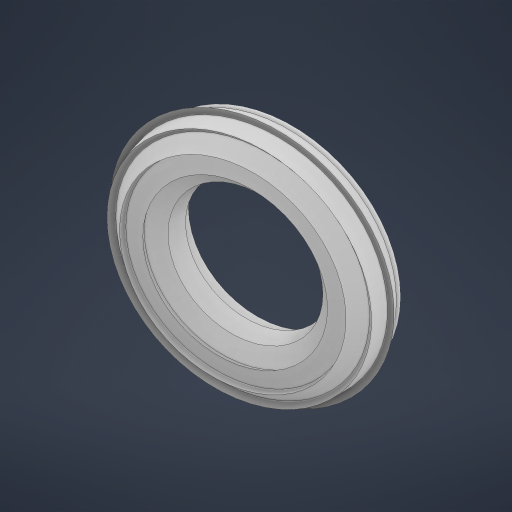
# Autodesk Inventor part: coba
Saved by Autodesk Inventor 2024.3 (Build 283343000, 343)
## iProperties
Created: 2025-06-21
Part Number: coba
Material: Generic
Document SubType Name: Modeling
Designer: Akbar Syihabuddin
Density: 1 g/cm^3
Appearance: Default
Author: Akbar Syihabuddin
Autodesk Inventor part; units mm, degrees
ref_plane "YZ Plane" through (0, 0, 0) normal (1, 0, 0) x (0, 1, 0)
ref_plane "XZ Plane" through (0, 0, 0) normal (0, 1, 0) x (-1, 0, 0)
ref_plane "XY Plane" through (0, 0, 0) normal (0, 0, 1) x (1, 0, 0)
sketch "Sketch1" plane through (0, 0, 0) normal (0, 1, 0) x (-1, 0, 0)
  line L0 (0, 1270.9169) -> (0, 1070.9169)
  line L1 (0, 1070.9169) -> (280.5773, 1070.9169)
  circle A0 centre (280.5773, 1070.9169) radius 150
  arc A1 (0, 862.6395) -> (280.5773, 1070.9169) centre (285.6481, 770.9597) ccw
  line L2 (0, 1671.4874) -> (1000, 1671.4874)
  line L3 (1000, 1671.4874) -> (1000, 2371.4874)
  line L4 (1000, 2371.4874) -> (0, 2371.4874)
  line L5 (0, 2371.4874) -> (0, 1671.4874)
  line L6 (663.7557, 3727.8622) -> (677.7261, 3727.8622) construction
  line L7 (677.7261, 3727.8622) -> (677.7261, 3724.6141) construction
  line L8 (677.7261, 3724.6141) -> (663.7557, 3724.6141) construction
  line L9 (663.7557, 3724.6141) -> (663.7557, 3727.8622) construction
  line L10 (500, 2021.4874) -> (1196.7714, 1270.9169)
  line L11 (1196.7714, 1270.9169) -> (1168.0077, -285.8687)
  line L12 (1168.0077, -285.8687) -> (464.4615, -168.1988)
  line L13 (464.4615, -168.1988) -> (320.7847, -408.7683)
  line L14 (1361.4266, 1423.77) -> (-428.0148, 1423.77)
  line L15 (-500, 1671.4874) -> (-500, 2371.4874)
  line L16 (-500, 2371.4874) -> (-1500, 2371.4874)
  line L17 (-1500, 2371.4874) -> (-1500, 1671.4874)
  line L18 (-1500, 1671.4874) -> (-500, 1671.4874)
  line L19 (2500, 1671.4874) -> (2500, 2371.4874)
  line L20 (2500, 2371.4874) -> (1500, 2371.4874)
  line L21 (1500, 2371.4874) -> (1500, 1671.4874)
  line L22 (1500, 1671.4874) -> (2500, 1671.4874)
  line L23 (1000, 1671.4874) -> (1000, 2371.4874)
  line L24 (1000, 2371.4874) -> (0, 2371.4874)
  line L25 (0, 2371.4874) -> (0, 1671.4874)
  line L26 (0, 1671.4874) -> (1000, 1671.4874)
  line L27 (500, 2021.4874) -> (500, -515.8022)
  line L28 (1000, 871.4874) -> (0, 871.4874)
  line L29 (1000, 871.4874) -> (0, 871.4874)
  line L30 (1000, 171.4874) -> (1000, 871.4874)
  line L31 (1000, 171.4874) -> (1000, 871.4874)
  line L32 (0, 871.4874) -> (0, 171.4874)
  line L33 (0, 871.4874) -> (0, 171.4874)
  line L34 (0, 171.4874) -> (1000, 171.4874)
  line L35 (0, 171.4874) -> (1000, 171.4874)
  line L36 (1000, -628.5126) -> (0, -628.5126)
  line L37 (1000, -628.5126) -> (0, -628.5126)
  line L38 (1000, -1328.5126) -> (1000, -628.5126)
  line L39 (1000, -1328.5126) -> (1000, -628.5126)
  line L40 (0, -628.5126) -> (0, -1328.5126)
  line L41 (0, -628.5126) -> (0, -1328.5126)
  line L42 (0, -1328.5126) -> (1000, -1328.5126)
  line L43 (0, -1328.5126) -> (1000, -1328.5126)
  line L44 (1000, -2128.5126) -> (0, -2128.5126)
  line L45 (1000, -2128.5126) -> (0, -2128.5126)
  line L46 (1000, -2828.5126) -> (1000, -2128.5126)
  line L47 (1000, -2828.5126) -> (1000, -2128.5126)
  line L48 (0, -2128.5126) -> (0, -2828.5126)
  line L49 (0, -2128.5126) -> (0, -2828.5126)
  line L50 (0, -2828.5126) -> (1000, -2828.5126)
  line L51 (0, -2828.5126) -> (1000, -2828.5126)
  line L52 (1000, -3628.5126) -> (0, -3628.5126)
  line L53 (1000, -3628.5126) -> (0, -3628.5126)
  line L54 (1000, -4328.5126) -> (1000, -3628.5126)
  line L55 (1000, -4328.5126) -> (1000, -3628.5126)
  line L56 (0, -3628.5126) -> (0, -4328.5126)
  line L57 (0, -3628.5126) -> (0, -4328.5126)
  line L58 (0, -4328.5126) -> (1000, -4328.5126)
  line L59 (0, -4328.5126) -> (1000, -4328.5126)
  line L60 (1000, -5128.5126) -> (0, -5128.5126)
  line L61 (1000, -5128.5126) -> (0, -5128.5126)
  line L62 (1000, -5828.5126) -> (1000, -5128.5126)
  line L63 (1000, -5828.5126) -> (1000, -5128.5126)
  line L64 (0, -5128.5126) -> (0, -5828.5126)
  line L65 (0, -5128.5126) -> (0, -5828.5126)
  line L66 (0, -5828.5126) -> (1000, -5828.5126)
  line L67 (0, -5828.5126) -> (1000, -5828.5126)
  line L68 (1000, -6628.5126) -> (0, -6628.5126)
  line L69 (1000, -6628.5126) -> (0, -6628.5126)
  line L70 (1000, -7328.5126) -> (1000, -6628.5126)
  line L71 (1000, -7328.5126) -> (1000, -6628.5126)
  line L72 (0, -6628.5126) -> (0, -7328.5126)
  line L73 (0, -6628.5126) -> (0, -7328.5126)
  line L74 (0, -7328.5126) -> (1000, -7328.5126)
  line L75 (0, -7328.5126) -> (1000, -7328.5126)
  line L76 (1000, -8128.5126) -> (0, -8128.5126)
  line L77 (1000, -8128.5126) -> (0, -8128.5126)
  line L78 (1000, -8828.5126) -> (1000, -8128.5126)
  line L79 (1000, -8828.5126) -> (1000, -8128.5126)
  line L80 (0, -8128.5126) -> (0, -8828.5126)
  line L81 (0, -8128.5126) -> (0, -8828.5126)
  line L82 (0, -8828.5126) -> (1000, -8828.5126)
  line L83 (0, -8828.5126) -> (1000, -8828.5126)
  line L84 (1000, -9628.5126) -> (0, -9628.5126)
  line L85 (1000, -9628.5126) -> (0, -9628.5126)
  line L86 (1000, -10328.5126) -> (1000, -9628.5126)
  line L87 (1000, -10328.5126) -> (1000, -9628.5126)
  line L88 (0, -9628.5126) -> (0, -10328.5126)
  line L89 (0, -9628.5126) -> (0, -10328.5126)
  line L90 (0, -10328.5126) -> (1000, -10328.5126)
  line L91 (0, -10328.5126) -> (1000, -10328.5126)
  line L92 (1000, -11128.5126) -> (0, -11128.5126)
  line L93 (1000, -11128.5126) -> (0, -11128.5126)
  line L94 (1000, -11828.5126) -> (1000, -11128.5126)
  line L95 (1000, -11828.5126) -> (1000, -11128.5126)
  line L96 (0, -11128.5126) -> (0, -11828.5126)
  line L97 (0, -11128.5126) -> (0, -11828.5126)
  line L98 (0, -11828.5126) -> (1000, -11828.5126)
  line L99 (0, -11828.5126) -> (1000, -11828.5126)
  line L100 (1000, -12628.5126) -> (0, -12628.5126)
  line L101 (1000, -12628.5126) -> (0, -12628.5126)
  line L102 (1000, -13328.5126) -> (1000, -12628.5126)
  line L103 (1000, -13328.5126) -> (1000, -12628.5126)
  line L104 (0, -12628.5126) -> (0, -13328.5126)
  line L105 (0, -12628.5126) -> (0, -13328.5126)
  line L106 (0, -13328.5126) -> (1000, -13328.5126)
  line L107 (0, -13328.5126) -> (1000, -13328.5126)
  line L108 (1000, -14128.5126) -> (0, -14128.5126)
  line L109 (1000, -14128.5126) -> (0, -14128.5126)
  line L110 (1000, -14828.5126) -> (1000, -14128.5126)
  line L111 (1000, -14828.5126) -> (1000, -14128.5126)
  line L112 (0, -14128.5126) -> (0, -14828.5126)
  line L113 (0, -14128.5126) -> (0, -14828.5126)
  line L114 (0, -14828.5126) -> (1000, -14828.5126)
  line L115 (0, -14828.5126) -> (1000, -14828.5126)
  line L116 (1000, -15628.5126) -> (0, -15628.5126)
  line L117 (1000, -15628.5126) -> (0, -15628.5126)
  line L118 (1000, -16328.5126) -> (1000, -15628.5126)
  line L119 (1000, -16328.5126) -> (1000, -15628.5126)
  line L120 (0, -15628.5126) -> (0, -16328.5126)
  line L121 (0, -15628.5126) -> (0, -16328.5126)
  line L122 (0, -16328.5126) -> (1000, -16328.5126)
  line L123 (0, -16328.5126) -> (1000, -16328.5126)
  line L124 (1000, -17128.5126) -> (0, -17128.5126)
  line L125 (1000, -17128.5126) -> (0, -17128.5126)
  line L126 (1000, -17828.5126) -> (1000, -17128.5126)
  line L127 (1000, -17828.5126) -> (1000, -17128.5126)
  line L128 (0, -17128.5126) -> (0, -17828.5126)
  line L129 (0, -17128.5126) -> (0, -17828.5126)
  line L130 (0, -17828.5126) -> (1000, -17828.5126)
  line L131 (0, -17828.5126) -> (1000, -17828.5126)
  line L132 (1000, -18628.5126) -> (0, -18628.5126)
  line L133 (1000, -18628.5126) -> (0, -18628.5126)
  line L134 (1000, -19328.5126) -> (1000, -18628.5126)
  line L135 (1000, -19328.5126) -> (1000, -18628.5126)
  line L136 (0, -18628.5126) -> (0, -19328.5126)
  line L137 (0, -18628.5126) -> (0, -19328.5126)
  line L138 (0, -19328.5126) -> (1000, -19328.5126)
  line L139 (0, -19328.5126) -> (1000, -19328.5126)
  line L140 (1000, -20128.5126) -> (0, -20128.5126)
  line L141 (1000, -20128.5126) -> (0, -20128.5126)
  line L142 (1000, -20828.5126) -> (1000, -20128.5126)
  line L143 (1000, -20828.5126) -> (1000, -20128.5126)
  line L144 (0, -20128.5126) -> (0, -20828.5126)
  line L145 (0, -20128.5126) -> (0, -20828.5126)
  line L146 (0, -20828.5126) -> (1000, -20828.5126)
  line L147 (0, -20828.5126) -> (1000, -20828.5126)
  line L148 (1000, -21628.5126) -> (0, -21628.5126)
  line L149 (1000, -21628.5126) -> (0, -21628.5126)
  line L150 (1000, -22328.5126) -> (1000, -21628.5126)
  line L151 (1000, -22328.5126) -> (1000, -21628.5126)
  line L152 (0, -21628.5126) -> (0, -22328.5126)
  line L153 (0, -21628.5126) -> (0, -22328.5126)
  line L154 (0, -22328.5126) -> (1000, -22328.5126)
  line L155 (0, -22328.5126) -> (1000, -22328.5126)
  line L156 (1000, -23128.5126) -> (0, -23128.5126)
  line L157 (1000, -23128.5126) -> (0, -23128.5126)
  line L158 (1000, -23828.5126) -> (1000, -23128.5126)
  line L159 (1000, -23828.5126) -> (1000, -23128.5126)
  line L160 (0, -23128.5126) -> (0, -23828.5126)
  line L161 (0, -23128.5126) -> (0, -23828.5126)
  line L162 (0, -23828.5126) -> (1000, -23828.5126)
  line L163 (0, -23828.5126) -> (1000, -23828.5126)
  line L164 (1000, -24628.5126) -> (0, -24628.5126)
  line L165 (1000, -24628.5126) -> (0, -24628.5126)
  line L166 (1000, -25328.5126) -> (1000, -24628.5126)
  line L167 (1000, -25328.5126) -> (1000, -24628.5126)
  line L168 (0, -24628.5126) -> (0, -25328.5126)
  line L169 (0, -24628.5126) -> (0, -25328.5126)
  line L170 (0, -25328.5126) -> (1000, -25328.5126)
  line L171 (0, -25328.5126) -> (1000, -25328.5126)
  line L172 (1000, -26128.5126) -> (0, -26128.5126)
  line L173 (1000, -26128.5126) -> (0, -26128.5126)
  line L174 (1000, -26828.5126) -> (1000, -26128.5126)
  line L175 (1000, -26828.5126) -> (1000, -26128.5126)
  line L176 (0, -26128.5126) -> (0, -26828.5126)
  line L177 (0, -26128.5126) -> (0, -26828.5126)
  line L178 (0, -26828.5126) -> (1000, -26828.5126)
  line L179 (0, -26828.5126) -> (1000, -26828.5126)
  line L180 (1000, -27628.5126) -> (0, -27628.5126)
  line L181 (1000, -27628.5126) -> (0, -27628.5126)
  line L182 (1000, -28328.5126) -> (1000, -27628.5126)
  line L183 (1000, -28328.5126) -> (1000, -27628.5126)
  line L184 (0, -27628.5126) -> (0, -28328.5126)
  line L185 (0, -27628.5126) -> (0, -28328.5126)
  line L186 (0, -28328.5126) -> (1000, -28328.5126)
  line L187 (0, -28328.5126) -> (1000, -28328.5126)
  line L188 (1000, -29128.5126) -> (0, -29128.5126)
  line L189 (1000, -29128.5126) -> (0, -29128.5126)
  line L190 (1000, -29828.5126) -> (1000, -29128.5126)
  line L191 (1000, -29828.5126) -> (1000, -29128.5126)
  line L192 (0, -29128.5126) -> (0, -29828.5126)
  line L193 (0, -29128.5126) -> (0, -29828.5126)
  line L194 (0, -29828.5126) -> (1000, -29828.5126)
  line L195 (0, -29828.5126) -> (1000, -29828.5126)
  line L196 (1000, -30628.5126) -> (0, -30628.5126)
  line L197 (1000, -30628.5126) -> (0, -30628.5126)
  line L198 (1000, -31328.5126) -> (1000, -30628.5126)
  line L199 (1000, -31328.5126) -> (1000, -30628.5126)
  line L200 (0, -30628.5126) -> (0, -31328.5126)
  line L201 (0, -30628.5126) -> (0, -31328.5126)
  line L202 (0, -31328.5126) -> (1000, -31328.5126)
  line L203 (0, -31328.5126) -> (1000, -31328.5126)
  line L204 (1000, -32128.5126) -> (0, -32128.5126)
  line L205 (1000, -32128.5126) -> (0, -32128.5126)
  line L206 (1000, -32828.5126) -> (1000, -32128.5126)
  line L207 (1000, -32828.5126) -> (1000, -32128.5126)
  line L208 (0, -32128.5126) -> (0, -32828.5126)
  line L209 (0, -32128.5126) -> (0, -32828.5126)
  line L210 (0, -32828.5126) -> (1000, -32828.5126)
  line L211 (0, -32828.5126) -> (1000, -32828.5126)
  line L212 (1000, -33628.5126) -> (0, -33628.5126)
  line L213 (1000, -33628.5126) -> (0, -33628.5126)
  line L214 (1000, -34328.5126) -> (1000, -33628.5126)
  line L215 (1000, -34328.5126) -> (1000, -33628.5126)
  line L216 (0, -33628.5126) -> (0, -34328.5126)
  line L217 (0, -33628.5126) -> (0, -34328.5126)
  line L218 (0, -34328.5126) -> (1000, -34328.5126)
  line L219 (0, -34328.5126) -> (1000, -34328.5126)
  line L220 (1000, -35128.5126) -> (0, -35128.5126)
  line L221 (1000, -35128.5126) -> (0, -35128.5126)
  line L222 (1000, -35828.5126) -> (1000, -35128.5126)
  line L223 (1000, -35828.5126) -> (1000, -35128.5126)
  line L224 (0, -35128.5126) -> (0, -35828.5126)
  line L225 (0, -35128.5126) -> (0, -35828.5126)
  line L226 (0, -35828.5126) -> (1000, -35828.5126)
  line L227 (0, -35828.5126) -> (1000, -35828.5126)
  line L228 (1000, -36628.5126) -> (0, -36628.5126)
  line L229 (1000, -36628.5126) -> (0, -36628.5126)
  line L230 (1000, -37328.5126) -> (1000, -36628.5126)
  line L231 (1000, -37328.5126) -> (1000, -36628.5126)
  line L232 (0, -36628.5126) -> (0, -37328.5126)
  line L233 (0, -36628.5126) -> (0, -37328.5126)
  line L234 (0, -37328.5126) -> (1000, -37328.5126)
  line L235 (0, -37328.5126) -> (1000, -37328.5126)
  line L236 (1000, -38128.5126) -> (0, -38128.5126)
  line L237 (1000, -38128.5126) -> (0, -38128.5126)
  line L238 (1000, -38828.5126) -> (1000, -38128.5126)
  line L239 (1000, -38828.5126) -> (1000, -38128.5126)
  line L240 (0, -38128.5126) -> (0, -38828.5126)
  line L241 (0, -38128.5126) -> (0, -38828.5126)
  line L242 (0, -38828.5126) -> (1000, -38828.5126)
  line L243 (0, -38828.5126) -> (1000, -38828.5126)
  line L244 (1000, -39628.5126) -> (0, -39628.5126)
  line L245 (1000, -39628.5126) -> (0, -39628.5126)
  line L246 (1000, -40328.5126) -> (1000, -39628.5126)
  line L247 (1000, -40328.5126) -> (1000, -39628.5126)
  line L248 (0, -39628.5126) -> (0, -40328.5126)
  line L249 (0, -39628.5126) -> (0, -40328.5126)
  line L250 (0, -40328.5126) -> (1000, -40328.5126)
  line L251 (0, -40328.5126) -> (1000, -40328.5126)
  line L252 (1000, -41128.5126) -> (0, -41128.5126)
  line L253 (1000, -41128.5126) -> (0, -41128.5126)
  line L254 (1000, -41828.5126) -> (1000, -41128.5126)
  line L255 (1000, -41828.5126) -> (1000, -41128.5126)
  line L256 (0, -41128.5126) -> (0, -41828.5126)
  line L257 (0, -41128.5126) -> (0, -41828.5126)
  line L258 (0, -41828.5126) -> (1000, -41828.5126)
  line L259 (0, -41828.5126) -> (1000, -41828.5126)
  circle A2 centre (1648.4251, 5737.6204) radius 272.6746
  line L260 (1594.4602, 7563.1402) -> (599.9131, 7563.1402)
  line L261 (599.9131, 7563.1402) -> (599.9131, 6816.0626)
  line L262 (599.9131, 6816.0626) -> (1594.4602, 6816.0626)
  line L263 (1594.4602, 6816.0626) -> (1594.4602, 7563.1402)
  line L264 (166.2687, 5993.7986) -> (970.8742, 6578.3787)
  line L265 (-272.8525, 6598.197) -> (166.2687, 5993.7986)
  line L266 (531.753, 7182.7771) -> (-272.8525, 6598.197)
  line L267 (970.8742, 6578.3787) -> (531.753, 7182.7771)
  line L268 (298.7576, 5073.6832) -> (606.0896, 6019.5536)
  line L269 (-411.7554, 5304.5428) -> (298.7576, 5073.6832)
  line L270 (-104.4234, 6250.4133) -> (-411.7554, 5304.5428)
  line L271 (606.0896, 6019.5536) -> (-104.4234, 6250.4133)
  line L272 (946.7737, 4407.1692) -> (639.4417, 5353.0397)
  line L273 (236.2607, 4176.3096) -> (946.7737, 4407.1692)
  line L274 (-71.0712, 5122.18) -> (236.2607, 4176.3096)
  line L275 (639.4417, 5353.0397) -> (-71.0712, 5122.18)
  line L276 (1862.7967, 4248.8424) -> (1058.1913, 4833.4225)
  line L277 (1423.6756, 3644.444) -> (1862.7967, 4248.8424)
  line L278 (619.0701, 4229.0241) -> (1423.6756, 3644.444)
  line L279 (1058.1913, 4833.4225) -> (619.0701, 4229.0241)
  line L280 (2696.9371, 4659.1782) -> (1702.3901, 4659.1782)
  line L281 (2696.9371, 3912.1006) -> (2696.9371, 4659.1782)
  line L282 (1702.3901, 3912.1006) -> (2696.9371, 3912.1006)
  line L283 (1702.3901, 4659.1782) -> (1702.3901, 3912.1006)
  line L284 (3130.5816, 5481.4422) -> (2325.9761, 4896.8621)
  line L285 (3569.7028, 4877.0438) -> (3130.5816, 5481.4422)
  line L286 (2765.0973, 4292.4637) -> (3569.7028, 4877.0438)
  line L287 (2325.9761, 4896.8621) -> (2765.0973, 4292.4637)
  line L288 (2998.0927, 6401.5576) -> (2690.7607, 5455.6871)
  line L289 (3708.6056, 6170.6979) -> (2998.0927, 6401.5576)
  line L290 (3401.2737, 5224.8275) -> (3708.6056, 6170.6979)
  line L291 (2690.7607, 5455.6871) -> (3401.2737, 5224.8275)
  line L292 (2350.0766, 7068.0715) -> (2657.4085, 6122.2011)
  line L293 (3060.5896, 7298.9312) -> (2350.0766, 7068.0715)
  line L294 (3367.9215, 6353.0607) -> (3060.5896, 7298.9312)
  line L295 (2657.4085, 6122.2011) -> (3367.9215, 6353.0607)
  line L296 (1434.0535, 7226.3984) -> (2238.659, 6641.8183)
  line L297 (1873.1747, 7830.7968) -> (1434.0535, 7226.3984)
  line L298 (2677.7802, 7246.2167) -> (1873.1747, 7830.7968)
  line L299 (2238.659, 6641.8183) -> (2677.7802, 7246.2167)
  line L300 (7155.2972, -58.1035) -> (-4493.949, -58.1035)
  line L301 (7155.2972, -58.1035) -> (8996.4598, -9718.9767)
  circle A3 centre (17696.4177, 10411.0259) radius 272.6746
  line L302 (17750.3826, 12236.5457) -> (18744.9297, 12236.5457)
  line L303 (18744.9297, 12236.5457) -> (18744.9297, 11489.4681)
  line L304 (18744.9297, 11489.4681) -> (17750.3826, 11489.4681)
  line L305 (17750.3826, 11489.4681) -> (17750.3826, 12236.5457)
  line L306 (19178.5741, 10667.2041) -> (18373.9687, 11251.7842)
  line L307 (19617.6953, 11271.6025) -> (19178.5741, 10667.2041)
  line L308 (18813.0898, 11856.1826) -> (19617.6953, 11271.6025)
  line L309 (18373.9687, 11251.7842) -> (18813.0898, 11856.1826)
  line L310 (19046.0852, 9747.0887) -> (18738.7532, 10692.9592)
  line L311 (19756.5982, 9977.9484) -> (19046.0852, 9747.0887)
  line L312 (19449.2662, 10923.8188) -> (19756.5982, 9977.9484)
  line L313 (18738.7532, 10692.9592) -> (19449.2662, 10923.8188)
  line L314 (18398.0691, 9080.5748) -> (18705.4011, 10026.4452)
  line L315 (19108.5821, 8849.7151) -> (18398.0691, 9080.5748)
  line L316 (19415.914, 9795.5856) -> (19108.5821, 8849.7151)
  line L317 (18705.4011, 10026.4452) -> (19415.914, 9795.5856)
  line L318 (17482.0461, 8922.248) -> (18286.6515, 9506.828)
  line L319 (17921.1672, 8317.8495) -> (17482.0461, 8922.248)
  line L320 (18725.7727, 8902.4296) -> (17921.1672, 8317.8495)
  line L321 (18286.6515, 9506.828) -> (18725.7727, 8902.4296)
  line L322 (16647.9057, 9332.5837) -> (17642.4527, 9332.5837)
  line L323 (16647.9057, 8585.5061) -> (16647.9057, 9332.5837)
  line L324 (17642.4527, 8585.5061) -> (16647.9057, 8585.5061)
  line L325 (17642.4527, 9332.5837) -> (17642.4527, 8585.5061)
  line L326 (16214.2612, 10154.8477) -> (17018.8667, 9570.2676)
  line L327 (15775.14, 9550.4493) -> (16214.2612, 10154.8477)
  line L328 (16579.7455, 8965.8692) -> (15775.14, 9550.4493)
  line L329 (17018.8667, 9570.2676) -> (16579.7455, 8965.8692)
  line L330 (16346.7501, 11074.9631) -> (16654.0821, 10129.0927)
  line L331 (15636.2372, 10844.1035) -> (16346.7501, 11074.9631)
  line L332 (15943.5691, 9898.233) -> (15636.2372, 10844.1035)
  line L333 (16654.0821, 10129.0927) -> (15943.5691, 9898.233)
  line L334 (16994.7662, 11741.4771) -> (16687.4343, 10795.6066)
  line L335 (16284.2532, 11972.3367) -> (16994.7662, 11741.4771)
  line L336 (15976.9213, 11026.4663) -> (16284.2532, 11972.3367)
  line L337 (16687.4343, 10795.6066) -> (15976.9213, 11026.4663)
  line L338 (17910.7893, 11899.8039) -> (17106.1838, 11315.2238)
  line L339 (17471.6681, 12504.2023) -> (17910.7893, 11899.8039)
  line L340 (16667.0626, 11919.6222) -> (17471.6681, 12504.2023)
  line L341 (17106.1838, 11315.2238) -> (16667.0626, 11919.6222)
  circle A4 centre (1648.4251, -5853.8275) radius 272.6746
  line L342 (1594.4602, -7679.3472) -> (599.9131, -7679.3472)
  line L343 (599.9131, -7679.3472) -> (599.9131, -6932.2697)
  line L344 (599.9131, -6932.2697) -> (1594.4602, -6932.2697)
  line L345 (1594.4602, -6932.2697) -> (1594.4602, -7679.3472)
  line L346 (166.2687, -6110.0056) -> (970.8742, -6694.5857)
  line L347 (-272.8525, -6714.4041) -> (166.2687, -6110.0056)
  line L348 (531.753, -7298.9842) -> (-272.8525, -6714.4041)
  line L349 (970.8742, -6694.5857) -> (531.753, -7298.9842)
  line L350 (298.7576, -5189.8903) -> (606.0896, -6135.7607)
  line L351 (-411.7554, -5420.7499) -> (298.7576, -5189.8903)
  line L352 (-104.4234, -6366.6204) -> (-411.7554, -5420.7499)
  line L353 (606.0896, -6135.7607) -> (-104.4234, -6366.6204)
  line L354 (946.7737, -4523.3763) -> (639.4417, -5469.2468)
  line L355 (236.2607, -4292.5167) -> (946.7737, -4523.3763)
  line L356 (-71.0712, -5238.3871) -> (236.2607, -4292.5167)
  line L357 (639.4417, -5469.2468) -> (-71.0712, -5238.3871)
  line L358 (1862.7967, -4365.0495) -> (1058.1913, -4949.6296)
  line L359 (1423.6756, -3760.651) -> (1862.7967, -4365.0495)
  line L360 (619.0701, -4345.2311) -> (1423.6756, -3760.651)
  line L361 (1058.1913, -4949.6296) -> (619.0701, -4345.2311)
  line L362 (2696.9371, -4775.3852) -> (1702.3901, -4775.3852)
  line L363 (2696.9371, -4028.3077) -> (2696.9371, -4775.3852)
  line L364 (1702.3901, -4028.3077) -> (2696.9371, -4028.3077)
  line L365 (1702.3901, -4775.3852) -> (1702.3901, -4028.3077)
  line L366 (3130.5816, -5597.6493) -> (2325.9761, -5013.0692)
  line L367 (3569.7028, -4993.2508) -> (3130.5816, -5597.6493)
  line L368 (2765.0973, -4408.6707) -> (3569.7028, -4993.2508)
  line L369 (2325.9761, -5013.0692) -> (2765.0973, -4408.6707)
  line L370 (2998.0927, -6517.7647) -> (2690.7607, -5571.8942)
  line L371 (3708.6056, -6286.905) -> (2998.0927, -6517.7647)
  line L372 (3401.2737, -5341.0345) -> (3708.6056, -6286.905)
  line L373 (2690.7607, -5571.8942) -> (3401.2737, -5341.0345)
  line L374 (2350.0766, -7184.2786) -> (2657.4085, -6238.4081)
  line L375 (3060.5896, -7415.1383) -> (2350.0766, -7184.2786)
  line L376 (3367.9215, -6469.2678) -> (3060.5896, -7415.1383)
  line L377 (2657.4085, -6238.4081) -> (3367.9215, -6469.2678)
  line L378 (1434.0535, -7342.6054) -> (2238.659, -6758.0253)
  line L379 (1873.1747, -7947.0039) -> (1434.0535, -7342.6054)
  line L380 (2677.7802, -7362.4238) -> (1873.1747, -7947.0039)
  line L381 (2238.659, -6758.0253) -> (2677.7802, -7362.4238)
  line L382 (12886.9187, -3760.651) -> (12447.7976, -4365.0495)
  line L383 (11613.6572, -4775.3852) -> (12608.2042, -4775.3852)
  line L384 (12608.2042, -4028.3077) -> (11613.6572, -4028.3077)
  line L385 (11613.6572, -4028.3077) -> (11613.6572, -4775.3852)
  line L386 (11545.497, -4408.6707) -> (10740.8915, -4993.2508)
  line L387 (11984.6182, -5013.0692) -> (11545.497, -4408.6707)
  line L388 (11312.5017, -6517.7647) -> (11619.8336, -5571.8942)
  line L389 (12716.1341, -7679.3472) -> (13710.6812, -7679.3472)
  line L390 (13710.6812, -7679.3472) -> (13710.6812, -6932.2697)
  line L391 (14722.3497, -5420.7499) -> (14011.8367, -5189.8903)
  line L392 (14011.8367, -5189.8903) -> (13704.5048, -6135.7607)
  line L393 (14415.0177, -6366.6204) -> (14722.3497, -5420.7499)
  line L394 (13704.5048, -6135.7607) -> (14415.0177, -6366.6204)
  line L395 (13710.6812, -6932.2697) -> (12716.1341, -6932.2697)
  line L396 (14583.4468, -6714.4041) -> (14144.3256, -6110.0056)
  line L397 (13339.7202, -6694.5857) -> (13778.8413, -7298.9842)
  line L398 (13778.8413, -7298.9842) -> (14583.4468, -6714.4041)
  line L399 (14144.3256, -6110.0056) -> (13339.7202, -6694.5857)
  line L400 (11619.8336, -5571.8942) -> (10909.3206, -5341.0345)
  line L401 (11180.0127, -5597.6493) -> (11984.6182, -5013.0692)
  line L402 (10740.8915, -4993.2508) -> (11180.0127, -5597.6493)
  line L403 (10909.3206, -5341.0345) -> (10601.9887, -6286.905)
  line L404 (11653.1858, -6238.4081) -> (10942.6728, -6469.2678)
  line L405 (10601.9887, -6286.905) -> (11312.5017, -6517.7647)
  circle A5 centre (12662.1692, -5853.8275) radius 272.6746
  line L406 (11960.5177, -7184.2786) -> (11653.1858, -6238.4081)
  line L407 (12071.9353, -6758.0253) -> (11632.8141, -7362.4238)
  line L408 (11250.0047, -7415.1383) -> (11960.5177, -7184.2786)
  line L409 (10942.6728, -6469.2678) -> (11250.0047, -7415.1383)
  line L410 (11632.8141, -7362.4238) -> (12437.4196, -7947.0039)
  line L411 (12716.1341, -6932.2697) -> (12716.1341, -7679.3472)
  line L412 (12437.4196, -7947.0039) -> (12876.5408, -7342.6054)
  line L413 (12876.5408, -7342.6054) -> (12071.9353, -6758.0253)
  line L414 (13671.1526, -5469.2468) -> (14381.6656, -5238.3871)
  line L415 (13363.8206, -4523.3763) -> (13671.1526, -5469.2468)
  line L416 (14381.6656, -5238.3871) -> (14074.3336, -4292.5167)
  line L417 (14074.3336, -4292.5167) -> (13363.8206, -4523.3763)
  line L418 (13252.403, -4949.6296) -> (13691.5242, -4345.2311)
  line L419 (12447.7976, -4365.0495) -> (13252.403, -4949.6296)
  line L420 (12608.2042, -4775.3852) -> (12608.2042, -4028.3077)
  line L421 (13691.5242, -4345.2311) -> (12886.9187, -3760.651)
  point P0 (0, 0)
  point P1 (-1000, 2021.4874)
  point P2 (2000, 2021.4874)
  point P3 (500, 521.4874)
  point P4 (500, 521.4874)
  point P5 (500, -978.5126)
  point P6 (500, -978.5126)
  point P7 (500, -2478.5126)
  point P8 (500, -2478.5126)
  point P9 (500, -3978.5126)
  point P10 (500, -3978.5126)
  point P11 (500, -5478.5126)
  point P12 (500, -5478.5126)
  point P13 (500, -6978.5126)
  point P14 (500, -6978.5126)
  point P15 (500, -8478.5126)
  point P16 (500, -8478.5126)
  point P17 (500, -9978.5126)
  point P18 (500, -9978.5126)
  point P19 (500, -11478.5126)
  point P20 (500, -11478.5126)
  point P21 (500, -12978.5126)
  point P22 (500, -12978.5126)
  point P23 (500, -14478.5126)
  point P24 (500, -14478.5126)
  point P25 (500, -15978.5126)
  point P26 (500, -15978.5126)
  point P27 (500, -17478.5126)
  point P28 (500, -17478.5126)
  point P29 (500, -18978.5126)
  point P30 (500, -18978.5126)
  point P31 (500, -20478.5126)
  point P32 (500, -20478.5126)
  point P33 (500, -21978.5126)
  point P34 (500, -21978.5126)
  point P35 (500, -23478.5126)
  point P36 (500, -23478.5126)
  point P37 (500, -24978.5126)
  point P38 (500, -24978.5126)
  point P39 (500, -26478.5126)
  point P40 (500, -26478.5126)
  point P41 (500, -27978.5126)
  point P42 (500, -27978.5126)
  point P43 (500, -29478.5126)
  point P44 (500, -29478.5126)
  point P45 (500, -30978.5126)
  point P46 (500, -30978.5126)
  point P47 (500, -32478.5126)
  point P48 (500, -32478.5126)
  point P49 (500, -33978.5126)
  point P50 (500, -33978.5126)
  point P51 (500, -35478.5126)
  point P52 (500, -35478.5126)
  point P53 (500, -36978.5126)
  point P54 (500, -36978.5126)
  point P55 (500, -38478.5126)
  point P56 (500, -38478.5126)
  point P57 (500, -39978.5126)
  point P58 (500, -39978.5126)
  point P59 (500, -41478.5126)
  point P60 (500, -41478.5126)
  point P61 (7155.2972, -9892.8557)
  point P62 (11899.2478, -6995.7093)
  point P63 (12716.1341, -7226.0632)
  point P64 (13512.4077, -6932.2697)
  point P65 (13983.919, -6226.5479)
  point P66 (13950.5668, -5378.4596)
  point P67 (13425.0905, -4711.9456)
  point P68 (12608.2042, -4481.5917)
  point P69 (11811.9307, -4775.3852)
  point P70 (11340.4194, -5481.107)
  point P71 (11373.7715, -6329.1953)
  dimension "d0" = 200
  dimension "d1" = 90
  dimension "d2" = 300
  dimension "d3" = 300
  dimension "d4" = 1000
  dimension "d5" = 700
  dimension "d8" = 1500
  dimension "d11" = 1500
  dimension "d16" = 1500
  dimension "d23" = 360
  constraints: 836 end point, 41 symmetric about line, 6 centre point, 6 horizontal, 4 parallel, 4 vertical, 2 perpendicular, 2 point on circle, 1 coincident, 633 other
  measures "d0" distance of L0.start L0.end
  measures "d1" angle of L1 L0
  measures "d2" diameter of A0
  measures "d3" radius of A1
  measures "d4" distance of L4.end L3.end
  measures "d5" distance of L3.end L2.end
  measures "d8" distance of L2.start L17.end
  measures "d11" distance of L2.start L21.end
  measures "d16" distance of L2.start L32.end
revolve "Revolution1" add sketch "Sketch1" angle 360 about axis through (-7155.2972, 0, -58.1035) along (-0.1872099, 0, -0.9823199) contours L419 L418 L415 L414 L392 L394 L399 L397 L395 L411 L413 L407 L406 L404 L388 L400 L401 L387 L383 L420
fillet "Fillet1" radius 200 1 edges at (-3074.0818, 0, -8305.7373)
chamfer "Chamfer1" distance 200 angle 45 1 edges at (-3772.1069, 0, -8788.5696)
body "Solid1"
